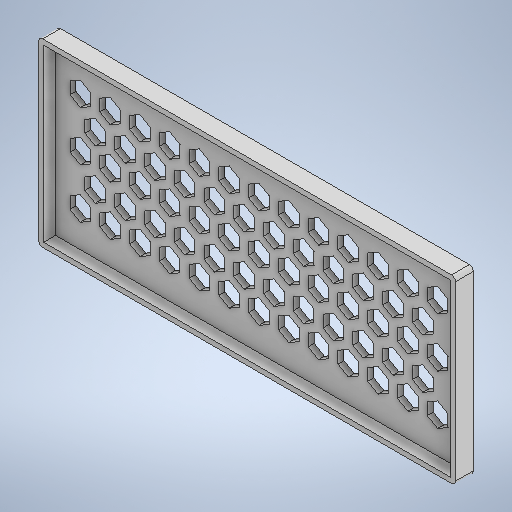
# Autodesk Inventor part: lm2596_box_lid_test
Saved by Autodesk Inventor 2025 (Build 290162000, 162)
## iProperties
Created: 2025-01-26
Part Number: lm2596_box_lid_test
Material: Všeobecné
Document SubType Name: Modeling
Designer: lukas
Density: 1 g/cm^3
Appearance: Výchozí
Author: lukas
## iProperties of the stored document lm2596_box_lid_3D tisk.ipt
Created: 2025-01-26
Part Number: lm2596_box_lid_3D tisk
Material: Všeobecné
Document SubType Name: Modeling
Designer: lukas
Density: 1 g/cm^3
Appearance: Výchozí
Author: lukas
Autodesk Inventor part; units mm, degrees
ref_plane "YZ Plane" through (0, 0, 0) normal (1, 0, 0) x (0, 1, 0)
ref_plane "XZ Plane" through (0, 0, 0) normal (0, 1, 0) x (-1, 0, 0)
ref_plane "XY Plane" through (0, 0, 0) normal (0, 0, 1) x (1, 0, 0)
sketch "Náčrt1" plane through (0, 0, 0) normal (0, 0, 1) x (1, 0, 0)
  line L0 (-105, 45.5) -> (105, 45.5)
  line L1 (105, 45.5) -> (105, -45.5)
  line L2 (105, -45.5) -> (-105, -45.5)
  line L3 (-105, -45.5) -> (-105, 45.5)
  line L4 (0, 63.7) -> (0, -63.7) projected
  line L5 (-147, 0) -> (147, 0) projected
  point P0 (0, 0)
  dimension "d0" = 210
  dimension "d1" = 91
  constraints: 8 end point, 2 parallel, 1 horizontal, 1 perpendicular, 2 other
  measures "d0" distance of L1.end L2.end
  measures "d1" distance of L0.end L1.end
extrude "Vysunutí1" add sketch "Náčrt1" along normal blind 3
sketch "Náčrt2" plane through (0, 0, 3) normal (0, 0, 1) x (1, 0, 0)
  line L0 (-105, 45.5) -> (-105, -45.5) projected
  line L1 (-105, -45.5) -> (105, -45.5) projected
  line L2 (105, -45.5) -> (105, 45.5) projected
  line L3 (105, 45.5) -> (-105, 45.5) projected
  line L4 (-164.5, 0) -> (164.5, 0) projected
  line L5 (0, -63.7) -> (0, 63.7) projected
  line L6 (-102.5, 43) -> (-102.5, -43)
  line L7 (-102.5, -43) -> (102.5, -43)
  line L8 (102.5, -43) -> (102.5, 43)
  line L9 (102.5, 43) -> (-102.5, 43)
  line L10 (-105, 45.5) -> (105, 45.5)
  line L11 (105, 45.5) -> (105, -45.5)
  line L12 (105, -45.5) -> (-105, -45.5)
  line L13 (-105, -45.5) -> (-105, 45.5)
  point P0 (0, 0)
  dimension "d5" = 2.5
  constraints: 16 end point, 2 parallel, 1 horizontal, 1 perpendicular, 3 other
  measures "d5" distance between parallel lines of L3 L9
extrude "Vysunutí2" add sketch "Náčrt2" along normal blind 6 contours L3 L5 L9 L6 L4 L0 | L4 L6 L7 L5 L1 L0 | L3 L2 L4 L8 L9 L5 | L5 L7 L8 L4 L2 L1
fillet "Zaoblení2" radius 2 4 edges at (105, -45.5, 4.5) (105, 45.5, 4.5) (-105, -45.5, 4.5) (-105, 45.5, 4.5)
sketch "Náčrt6" plane through (0, 0, 0) normal (0, 0, -1) x (-1, 0, 0)
  arc A0 (105, 43.5) -> (103, 45.5) centre (103, 43.5) ccw projected
  line L0 (-103, 45.5) -> (103, 45.5) projected
  arc A1 (-103, 45.5) -> (-105, 43.5) centre (-103, 43.5) ccw projected
  line L1 (-105, -43.5) -> (-105, 43.5) projected
  arc A2 (-105, -43.5) -> (-103, -45.5) centre (-103, -43.5) ccw projected
  line L2 (103, -45.5) -> (-103, -45.5) projected
  arc A3 (103, -45.5) -> (105, -43.5) centre (103, -43.5) ccw projected
  line L3 (105, 43.5) -> (105, -43.5) projected
  line L4 (0, -64.2799) -> (0, 64.2799) projected
  line L5 (-165.0799, 0) -> (165.0799, 0) projected
  line L6 (0, 6) -> (5.1962, 3)
  line L7 (5.1962, 3) -> (5.1962, -3)
  line L8 (5.1962, -3) -> (0, -6)
  line L9 (0, -6) -> (-5.1962, -3)
  line L10 (-5.1962, -3) -> (-5.1962, 3)
  line L11 (-5.1962, 3) -> (0, 6)
  line L12 (0, 0) -> (-2.5981, -4.5) construction
  line L13 (-7.5, -12.9904) -> (-10.0981, -17.4904) construction
  line L14 (-7.5, -18.9904) -> (-12.6962, -15.9904)
  line L15 (-12.6962, -15.9904) -> (-12.6962, -9.9904)
  line L16 (-2.3038, -9.9904) -> (-2.3038, -15.9904)
  line L17 (-12.6962, -9.9904) -> (-7.5, -6.9904)
  line L18 (-7.5, -6.9904) -> (-2.3038, -9.9904)
  line L19 (-2.3038, -15.9904) -> (-7.5, -18.9904)
  line L20 (-20.1962, 3) -> (-15, 6)
  line L21 (-15, 6) -> (-9.8038, 3)
  line L22 (-20.1962, -3) -> (-20.1962, 3)
  line L23 (-15, -6) -> (-20.1962, -3)
  line L24 (-9.8038, -3) -> (-15, -6)
  line L25 (-9.8038, 3) -> (-9.8038, -3)
  line L26 (9.8038, 3) -> (15, 6)
  line L27 (15, 6) -> (20.1962, 3)
  line L28 (9.8038, -3) -> (9.8038, 3)
  line L29 (15, -6) -> (9.8038, -3)
  line L30 (20.1962, -3) -> (15, -6)
  line L31 (20.1962, 3) -> (20.1962, -3)
  line L32 (-35.1962, 3) -> (-30, 6)
  line L33 (-30, 6) -> (-24.8038, 3)
  line L34 (-35.1962, -3) -> (-35.1962, 3)
  line L35 (-30, -6) -> (-35.1962, -3)
  line L36 (-24.8038, -3) -> (-30, -6)
  line L37 (-24.8038, 3) -> (-24.8038, -3)
  line L38 (24.8038, 3) -> (30, 6)
  line L39 (30, 6) -> (35.1962, 3)
  line L40 (24.8038, -3) -> (24.8038, 3)
  line L41 (30, -6) -> (24.8038, -3)
  line L42 (35.1962, -3) -> (30, -6)
  line L43 (35.1962, 3) -> (35.1962, -3)
  line L44 (-50.1962, 3) -> (-45, 6)
  line L45 (-45, 6) -> (-39.8038, 3)
  line L46 (-50.1962, -3) -> (-50.1962, 3)
  line L47 (-45, -6) -> (-50.1962, -3)
  line L48 (-39.8038, -3) -> (-45, -6)
  line L49 (-39.8038, 3) -> (-39.8038, -3)
  line L50 (39.8038, 3) -> (45, 6)
  line L51 (45, 6) -> (50.1962, 3)
  line L52 (39.8038, -3) -> (39.8038, 3)
  line L53 (45, -6) -> (39.8038, -3)
  line L54 (50.1962, -3) -> (45, -6)
  line L55 (50.1962, 3) -> (50.1962, -3)
  line L56 (-65.1962, 3) -> (-60, 6)
  line L57 (-60, 6) -> (-54.8038, 3)
  line L58 (-65.1962, -3) -> (-65.1962, 3)
  line L59 (-60, -6) -> (-65.1962, -3)
  line L60 (-54.8038, -3) -> (-60, -6)
  line L61 (-54.8038, 3) -> (-54.8038, -3)
  line L62 (54.8038, 3) -> (60, 6)
  line L63 (60, 6) -> (65.1962, 3)
  line L64 (54.8038, -3) -> (54.8038, 3)
  line L65 (60, -6) -> (54.8038, -3)
  line L66 (65.1962, -3) -> (60, -6)
  line L67 (65.1962, 3) -> (65.1962, -3)
  line L68 (-80.1962, 3) -> (-75, 6)
  line L69 (-75, 6) -> (-69.8038, 3)
  line L70 (-80.1962, -3) -> (-80.1962, 3)
  line L71 (-75, -6) -> (-80.1962, -3)
  line L72 (-69.8038, -3) -> (-75, -6)
  line L73 (-69.8038, 3) -> (-69.8038, -3)
  line L74 (69.8038, 3) -> (75, 6)
  line L75 (75, 6) -> (80.1962, 3)
  line L76 (69.8038, -3) -> (69.8038, 3)
  line L77 (75, -6) -> (69.8038, -3)
  line L78 (80.1962, -3) -> (75, -6)
  line L79 (80.1962, 3) -> (80.1962, -3)
  line L80 (-95.1962, 3) -> (-90, 6)
  line L81 (-90, 6) -> (-84.8038, 3)
  line L82 (-95.1962, -3) -> (-95.1962, 3)
  line L83 (-90, -6) -> (-95.1962, -3)
  line L84 (-84.8038, -3) -> (-90, -6)
  line L85 (-84.8038, 3) -> (-84.8038, -3)
  line L86 (84.8038, 3) -> (90, 6)
  line L87 (90, 6) -> (95.1962, 3)
  line L88 (84.8038, -3) -> (84.8038, 3)
  line L89 (90, -6) -> (84.8038, -3)
  line L90 (95.1962, -3) -> (90, -6)
  line L91 (95.1962, 3) -> (95.1962, -3)
  line L92 (7.5, -12.9904) -> (4.9019, -17.4904) construction
  line L93 (2.3038, -9.9904) -> (7.5, -6.9904)
  line L94 (2.3038, -15.9904) -> (2.3038, -9.9904)
  line L95 (7.5, -18.9904) -> (2.3038, -15.9904)
  line L96 (12.6962, -15.9904) -> (7.5, -18.9904)
  line L97 (7.5, -6.9904) -> (12.6962, -9.9904)
  line L98 (12.6962, -9.9904) -> (12.6962, -15.9904)
  line L99 (22.5, -12.9904) -> (19.9019, -17.4904) construction
  line L100 (17.3038, -9.9904) -> (22.5, -6.9904)
  line L101 (17.3038, -15.9904) -> (17.3038, -9.9904)
  line L102 (22.5, -18.9904) -> (17.3038, -15.9904)
  line L103 (27.6962, -15.9904) -> (22.5, -18.9904)
  line L104 (22.5, -6.9904) -> (27.6962, -9.9904)
  line L105 (27.6962, -9.9904) -> (27.6962, -15.9904)
  line L106 (37.5, -12.9904) -> (34.9019, -17.4904) construction
  line L107 (32.3038, -9.9904) -> (37.5, -6.9904)
  line L108 (32.3038, -15.9904) -> (32.3038, -9.9904)
  line L109 (37.5, -18.9904) -> (32.3038, -15.9904)
  line L110 (42.6962, -15.9904) -> (37.5, -18.9904)
  line L111 (37.5, -6.9904) -> (42.6962, -9.9904)
  line L112 (42.6962, -9.9904) -> (42.6962, -15.9904)
  line L113 (52.5, -12.9904) -> (49.9019, -17.4904) construction
  line L114 (47.3038, -9.9904) -> (52.5, -6.9904)
  line L115 (47.3038, -15.9904) -> (47.3038, -9.9904)
  line L116 (52.5, -18.9904) -> (47.3038, -15.9904)
  line L117 (57.6962, -15.9904) -> (52.5, -18.9904)
  line L118 (52.5, -6.9904) -> (57.6962, -9.9904)
  line L119 (57.6962, -9.9904) -> (57.6962, -15.9904)
  line L120 (67.5, -12.9904) -> (64.9019, -17.4904) construction
  line L121 (62.3038, -9.9904) -> (67.5, -6.9904)
  line L122 (62.3038, -15.9904) -> (62.3038, -9.9904)
  line L123 (67.5, -18.9904) -> (62.3038, -15.9904)
  line L124 (72.6962, -15.9904) -> (67.5, -18.9904)
  line L125 (67.5, -6.9904) -> (72.6962, -9.9904)
  line L126 (72.6962, -9.9904) -> (72.6962, -15.9904)
  line L127 (82.5, -12.9904) -> (79.9019, -17.4904) construction
  line L128 (77.3038, -9.9904) -> (82.5, -6.9904)
  line L129 (77.3038, -15.9904) -> (77.3038, -9.9904)
  line L130 (82.5, -18.9904) -> (77.3038, -15.9904)
  line L131 (87.6962, -15.9904) -> (82.5, -18.9904)
  line L132 (82.5, -6.9904) -> (87.6962, -9.9904)
  line L133 (87.6962, -9.9904) -> (87.6962, -15.9904)
  line L134 (-27.6962, -9.9904) -> (-22.5, -6.9904)
  line L135 (-22.5, -6.9904) -> (-17.3038, -9.9904)
  line L136 (-27.6962, -15.9904) -> (-27.6962, -9.9904)
  line L137 (-22.5, -12.9904) -> (-25.0981, -17.4904) construction
  line L138 (-22.5, -18.9904) -> (-27.6962, -15.9904)
  line L139 (-17.3038, -15.9904) -> (-22.5, -18.9904)
  line L140 (-17.3038, -9.9904) -> (-17.3038, -15.9904)
  line L141 (-42.6962, -9.9904) -> (-37.5, -6.9904)
  line L142 (-37.5, -6.9904) -> (-32.3038, -9.9904)
  line L143 (-42.6962, -15.9904) -> (-42.6962, -9.9904)
  line L144 (-37.5, -12.9904) -> (-40.0981, -17.4904) construction
  line L145 (-37.5, -18.9904) -> (-42.6962, -15.9904)
  line L146 (-32.3038, -15.9904) -> (-37.5, -18.9904)
  line L147 (-32.3038, -9.9904) -> (-32.3038, -15.9904)
  line L148 (-57.6962, -9.9904) -> (-52.5, -6.9904)
  line L149 (-52.5, -6.9904) -> (-47.3038, -9.9904)
  line L150 (-57.6962, -15.9904) -> (-57.6962, -9.9904)
  line L151 (-52.5, -12.9904) -> (-55.0981, -17.4904) construction
  line L152 (-52.5, -18.9904) -> (-57.6962, -15.9904)
  line L153 (-47.3038, -15.9904) -> (-52.5, -18.9904)
  line L154 (-47.3038, -9.9904) -> (-47.3038, -15.9904)
  line L155 (-72.6962, -9.9904) -> (-67.5, -6.9904)
  line L156 (-67.5, -6.9904) -> (-62.3038, -9.9904)
  line L157 (-72.6962, -15.9904) -> (-72.6962, -9.9904)
  line L158 (-67.5, -12.9904) -> (-70.0981, -17.4904) construction
  line L159 (-67.5, -18.9904) -> (-72.6962, -15.9904)
  line L160 (-62.3038, -15.9904) -> (-67.5, -18.9904)
  line L161 (-62.3038, -9.9904) -> (-62.3038, -15.9904)
  line L162 (-87.6962, -9.9904) -> (-82.5, -6.9904)
  line L163 (-82.5, -6.9904) -> (-77.3038, -9.9904)
  line L164 (-87.6962, -15.9904) -> (-87.6962, -9.9904)
  line L165 (-82.5, -12.9904) -> (-85.0981, -17.4904) construction
  line L166 (-82.5, -18.9904) -> (-87.6962, -15.9904)
  line L167 (-77.3038, -15.9904) -> (-82.5, -18.9904)
  line L168 (-77.3038, -9.9904) -> (-77.3038, -15.9904)
  line L169 (37.5, 18.0096) -> (42.6962, 15.0096)
  line L170 (32.3038, 15.0096) -> (37.5, 18.0096)
  line L171 (42.6962, 15.0096) -> (42.6962, 9.0096)
  line L172 (42.6962, 9.0096) -> (37.5, 6.0096)
  line L173 (37.5, 12.0096) -> (34.9019, 7.5096) construction
  line L174 (37.5, 6.0096) -> (32.3038, 9.0096)
  line L175 (32.3038, 9.0096) -> (32.3038, 15.0096)
  line L176 (-22.5, 18.0096) -> (-17.3038, 15.0096)
  line L177 (-12.6962, 15.0096) -> (-7.5, 18.0096)
  line L178 (-17.3038, 15.0096) -> (-17.3038, 9.0096)
  line L179 (-17.3038, 9.0096) -> (-22.5, 6.0096)
  line L180 (-7.5, 18.0096) -> (-2.3038, 15.0096)
  line L181 (-12.6962, 9.0096) -> (-12.6962, 15.0096)
  line L182 (-7.5, 12.0096) -> (-10.0981, 7.5096) construction
  line L183 (-7.5, 6.0096) -> (-12.6962, 9.0096)
  line L184 (-2.3038, 9.0096) -> (-7.5, 6.0096)
  line L185 (-2.3038, 15.0096) -> (-2.3038, 9.0096)
  line L186 (2.3038, 9.0096) -> (2.3038, 15.0096)
  line L187 (2.3038, 15.0096) -> (7.5, 18.0096)
  line L188 (7.5, 18.0096) -> (12.6962, 15.0096)
  line L189 (7.5, 12.0096) -> (4.9019, 7.5096) construction
  line L190 (12.6962, 9.0096) -> (7.5, 6.0096)
  line L191 (7.5, 6.0096) -> (2.3038, 9.0096)
  line L192 (22.5, 18.0096) -> (27.6962, 15.0096)
  line L193 (27.6962, 15.0096) -> (27.6962, 9.0096)
  line L194 (17.3038, 15.0096) -> (22.5, 18.0096)
  line L195 (27.6962, 9.0096) -> (22.5, 6.0096)
  line L196 (22.5, 12.0096) -> (19.9019, 7.5096) construction
  line L197 (22.5, 6.0096) -> (17.3038, 9.0096)
  line L198 (-57.6962, 9.0096) -> (-57.6962, 15.0096)
  line L199 (-52.5, 6.0096) -> (-57.6962, 9.0096)
  line L200 (-52.5, 12.0096) -> (-55.0981, 7.5096) construction
  line L201 (-57.6962, 15.0096) -> (-52.5, 18.0096)
  line L202 (12.6962, 15.0096) -> (12.6962, 9.0096)
  line L203 (17.3038, 9.0096) -> (17.3038, 15.0096)
  line L204 (52.5, 18.0096) -> (57.6962, 15.0096)
  line L205 (62.3038, 15.0096) -> (67.5, 18.0096)
  line L206 (62.3038, 9.0096) -> (62.3038, 15.0096)
  line L207 (67.5, 12.0096) -> (64.9019, 7.5096) construction
  line L208 (67.5, 6.0096) -> (62.3038, 9.0096)
  line L209 (47.3038, 15.0096) -> (52.5, 18.0096)
  line L210 (52.5, 12.0096) -> (49.9019, 7.5096) construction
  line L211 (57.6962, 9.0096) -> (52.5, 6.0096)
  line L212 (47.3038, 9.0096) -> (47.3038, 15.0096)
  line L213 (52.5, 6.0096) -> (47.3038, 9.0096)
  line L214 (57.6962, 15.0096) -> (57.6962, 9.0096)
  line L215 (67.5, 18.0096) -> (72.6962, 15.0096)
  line L216 (72.6962, 9.0096) -> (67.5, 6.0096)
  line L217 (77.3038, 15.0096) -> (82.5, 18.0096)
  line L218 (72.6962, 15.0096) -> (72.6962, 9.0096)
  line L219 (77.3038, 9.0096) -> (77.3038, 15.0096)
  line L220 (82.5, 18.0096) -> (87.6962, 15.0096)
  line L221 (82.5, 12.0096) -> (79.9019, 7.5096) construction
  line L222 (82.5, 6.0096) -> (77.3038, 9.0096)
  line L223 (87.6962, 15.0096) -> (87.6962, 9.0096)
  line L224 (87.6962, 9.0096) -> (82.5, 6.0096)
  line L225 (-22.5, 12.0096) -> (-25.0981, 7.5096) construction
  line L226 (-27.6962, 15.0096) -> (-22.5, 18.0096)
  line L227 (-22.5, 6.0096) -> (-27.6962, 9.0096)
  line L228 (-27.6962, 9.0096) -> (-27.6962, 15.0096)
  line L229 (-32.3038, 15.0096) -> (-32.3038, 9.0096)
  line L230 (-32.3038, 9.0096) -> (-37.5, 6.0096)
  line L231 (-37.5, 18.0096) -> (-32.3038, 15.0096)
  line L232 (-37.5, 12.0096) -> (-40.0981, 7.5096) construction
  line L233 (-42.6962, 15.0096) -> (-37.5, 18.0096)
  line L234 (-37.5, 6.0096) -> (-42.6962, 9.0096)
  line L235 (-42.6962, 9.0096) -> (-42.6962, 15.0096)
  line L236 (-47.3038, 15.0096) -> (-47.3038, 9.0096)
  line L237 (-47.3038, 9.0096) -> (-52.5, 6.0096)
  line L238 (-52.5, 18.0096) -> (-47.3038, 15.0096)
  line L239 (-82.5, 18.0096) -> (-77.3038, 15.0096)
  line L240 (-87.6962, 15.0096) -> (-82.5, 18.0096)
  line L241 (-77.3038, 9.0096) -> (-82.5, 6.0096)
  line L242 (-82.5, 12.0096) -> (-85.0981, 7.5096) construction
  line L243 (-87.6962, 9.0096) -> (-87.6962, 15.0096)
  line L244 (-82.5, 6.0096) -> (-87.6962, 9.0096)
  line L245 (-77.3038, 15.0096) -> (-77.3038, 9.0096)
  line L246 (-67.5, 18.0096) -> (-62.3038, 15.0096)
  line L247 (-62.3038, 15.0096) -> (-62.3038, 9.0096)
  line L248 (-72.6962, 15.0096) -> (-67.5, 18.0096)
  line L249 (-62.3038, 9.0096) -> (-67.5, 6.0096)
  line L250 (-67.5, 12.0096) -> (-70.0981, 7.5096) construction
  line L251 (-72.6962, 9.0096) -> (-72.6962, 15.0096)
  line L252 (-67.5, 6.0096) -> (-72.6962, 9.0096)
  line L253 (-45, 31) -> (-39.8038, 28)
  line L254 (-15, 19) -> (-20.1962, 22)
  line L255 (-20.1962, 28) -> (-15, 31)
  line L256 (-20.1962, 22) -> (-20.1962, 28)
  line L257 (-39.8038, 28) -> (-39.8038, 22)
  line L258 (-30, 31) -> (-24.8038, 28)
  line L259 (-35.1962, 22) -> (-35.1962, 28)
  line L260 (-24.8038, 28) -> (-24.8038, 22)
  line L261 (-24.8038, 22) -> (-30, 19)
  line L262 (-30, 19) -> (-35.1962, 22)
  line L263 (-35.1962, 28) -> (-30, 31)
  line L264 (-39.8038, 22) -> (-45, 19)
  line L265 (-45, 19) -> (-50.1962, 22)
  line L266 (-50.1962, 28) -> (-45, 31)
  line L267 (-50.1962, 22) -> (-50.1962, 28)
  line L268 (-65.1962, 28) -> (-60, 31)
  line L269 (-60, 31) -> (-54.8038, 28)
  line L270 (-65.1962, 22) -> (-65.1962, 28)
  line L271 (-54.8038, 22) -> (-60, 19)
  line L272 (-54.8038, 28) -> (-54.8038, 22)
  line L273 (-60, 19) -> (-65.1962, 22)
  line L274 (-80.1962, 28) -> (-75, 31)
  line L275 (-75, 31) -> (-69.8038, 28)
  line L276 (-80.1962, 22) -> (-80.1962, 28)
  line L277 (-69.8038, 28) -> (-69.8038, 22)
  line L278 (-69.8038, 22) -> (-75, 19)
  line L279 (-75, 19) -> (-80.1962, 22)
  line L280 (-84.8038, 28) -> (-84.8038, 22)
  line L281 (-90, 31) -> (-84.8038, 28)
  line L282 (-95.1962, 28) -> (-90, 31)
  line L283 (-95.1962, 22) -> (-95.1962, 28)
  line L284 (-84.8038, 22) -> (-90, 19)
  line L285 (-90, 19) -> (-95.1962, 22)
  line L286 (69.8038, 28) -> (75, 31)
  line L287 (69.8038, 22) -> (69.8038, 28)
  line L288 (60, 31) -> (65.1962, 28)
  line L289 (75, 19) -> (69.8038, 22)
  line L290 (65.1962, 28) -> (65.1962, 22)
  line L291 (54.8038, 28) -> (60, 31)
  line L292 (65.1962, 22) -> (60, 19)
  line L293 (54.8038, 22) -> (54.8038, 28)
  line L294 (50.1962, 28) -> (50.1962, 22)
  line L295 (35.1962, 22) -> (30, 19)
  line L296 (35.1962, 28) -> (35.1962, 22)
  line L297 (39.8038, 22) -> (39.8038, 28)
  line L298 (45, 19) -> (39.8038, 22)
  line L299 (-5.1962, 28) -> (0, 31)
  line L300 (-15, 31) -> (-9.8038, 28)
  line L301 (0, 31) -> (5.1962, 28)
  line L302 (-5.1962, 22) -> (-5.1962, 28)
  line L303 (-9.8038, 28) -> (-9.8038, 22)
  line L304 (-9.8038, 22) -> (-15, 19)
  line L305 (0, 25) -> (-2.5981, 20.5) construction
  line L306 (0, 19) -> (-5.1962, 22)
  line L307 (5.1962, 28) -> (5.1962, 22)
  line L308 (5.1962, 22) -> (0, 19)
  line L309 (9.8038, 28) -> (15, 31)
  line L310 (15, 31) -> (20.1962, 28)
  line L311 (24.8038, 22) -> (24.8038, 28)
  line L312 (24.8038, 28) -> (30, 31)
  line L313 (20.1962, 28) -> (20.1962, 22)
  line L314 (30, 31) -> (35.1962, 28)
  line L315 (39.8038, 28) -> (45, 31)
  line L316 (45, 31) -> (50.1962, 28)
  line L317 (50.1962, 22) -> (45, 19)
  line L318 (60, 19) -> (54.8038, 22)
  line L319 (80.1962, 22) -> (75, 19)
  line L320 (75, 31) -> (80.1962, 28)
  line L321 (90, 19) -> (84.8038, 22)
  line L322 (80.1962, 28) -> (80.1962, 22)
  line L323 (95.1962, 22) -> (90, 19)
  line L324 (84.8038, 22) -> (84.8038, 28)
  line L325 (84.8038, 28) -> (90, 31)
  line L326 (95.1962, 28) -> (95.1962, 22)
  line L327 (90, 31) -> (95.1962, 28)
  line L328 (9.8038, 22) -> (9.8038, 28)
  line L329 (15, 19) -> (9.8038, 22)
  line L330 (20.1962, 22) -> (15, 19)
  line L331 (30, 19) -> (24.8038, 22)
  line L332 (24.8038, -22) -> (30, -19)
  line L333 (15, -19) -> (20.1962, -22)
  line L334 (15, -31) -> (9.8038, -28)
  line L335 (9.8038, -28) -> (9.8038, -22)
  line L336 (9.8038, -22) -> (15, -19)
  line L337 (20.1962, -28) -> (15, -31)
  line L338 (20.1962, -22) -> (20.1962, -28)
  line L339 (24.8038, -28) -> (24.8038, -22)
  line L340 (30, -31) -> (24.8038, -28)
  line L341 (35.1962, -28) -> (30, -31)
  line L342 (39.8038, -28) -> (39.8038, -22)
  line L343 (39.8038, -22) -> (45, -19)
  line L344 (30, -19) -> (35.1962, -22)
  line L345 (35.1962, -22) -> (35.1962, -28)
  line L346 (45, -31) -> (39.8038, -28)
  line L347 (50.1962, -28) -> (45, -31)
  line L348 (50.1962, -22) -> (50.1962, -28)
  line L349 (54.8038, -22) -> (60, -19)
  line L350 (60, -19) -> (65.1962, -22)
  line L351 (75, -31) -> (69.8038, -28)
  line L352 (65.1962, -28) -> (60, -31)
  line L353 (69.8038, -28) -> (69.8038, -22)
  line L354 (65.1962, -22) -> (65.1962, -28)
  line L355 (54.8038, -28) -> (54.8038, -22)
  line L356 (60, -31) -> (54.8038, -28)
  line L357 (90, -31) -> (84.8038, -28)
  line L358 (95.1962, -28) -> (90, -31)
  line L359 (80.1962, -22) -> (80.1962, -28)
  line L360 (84.8038, -28) -> (84.8038, -22)
  line L361 (84.8038, -22) -> (90, -19)
  line L362 (95.1962, -22) -> (95.1962, -28)
  line L363 (90, -19) -> (95.1962, -22)
  line L364 (80.1962, -28) -> (75, -31)
  line L365 (75, -19) -> (80.1962, -22)
  line L366 (69.8038, -22) -> (75, -19)
  line L367 (45, -19) -> (50.1962, -22)
  line L368 (-50.1962, -22) -> (-45, -19)
  line L369 (-45, -19) -> (-39.8038, -22)
  line L370 (-54.8038, -22) -> (-54.8038, -28)
  line L371 (-50.1962, -28) -> (-50.1962, -22)
  line L372 (-39.8038, -22) -> (-39.8038, -28)
  line L373 (-45, -31) -> (-50.1962, -28)
  line L374 (-39.8038, -28) -> (-45, -31)
  line L375 (-65.1962, -28) -> (-65.1962, -22)
  line L376 (-80.1962, -22) -> (-75, -19)
  line L377 (-75, -19) -> (-69.8038, -22)
  line L378 (-69.8038, -22) -> (-69.8038, -28)
  line L379 (-69.8038, -28) -> (-75, -31)
  line L380 (-75, -31) -> (-80.1962, -28)
  line L381 (-80.1962, -28) -> (-80.1962, -22)
  line L382 (-65.1962, -22) -> (-60, -19)
  line L383 (-60, -19) -> (-54.8038, -22)
  line L384 (-95.1962, -22) -> (-90, -19)
  line L385 (-90, -19) -> (-84.8038, -22)
  line L386 (-95.1962, -28) -> (-95.1962, -22)
  line L387 (-90, -31) -> (-95.1962, -28)
  line L388 (-84.8038, -28) -> (-90, -31)
  line L389 (-84.8038, -22) -> (-84.8038, -28)
  line L390 (-54.8038, -28) -> (-60, -31)
  line L391 (-60, -31) -> (-65.1962, -28)
  line L392 (-24.8038, -28) -> (-30, -31)
  line L393 (-30, -31) -> (-35.1962, -28)
  line L394 (-20.1962, -22) -> (-15, -19)
  line L395 (-15, -31) -> (-20.1962, -28)
  line L396 (0, -19) -> (5.1962, -22)
  line L397 (5.1962, -22) -> (5.1962, -28)
  line L398 (0, -25) -> (-2.5981, -29.5) construction
  line L399 (5.1962, -28) -> (0, -31)
  line L400 (-5.1962, -28) -> (-5.1962, -22)
  line L401 (0, -31) -> (-5.1962, -28)
  line L402 (-5.1962, -22) -> (0, -19)
  line L403 (-9.8038, -22) -> (-9.8038, -28)
  line L404 (-9.8038, -28) -> (-15, -31)
  line L405 (-15, -19) -> (-9.8038, -22)
  line L406 (-20.1962, -28) -> (-20.1962, -22)
  line L407 (-24.8038, -22) -> (-24.8038, -28)
  line L408 (-30, -19) -> (-24.8038, -22)
  line L409 (-35.1962, -28) -> (-35.1962, -22)
  line L410 (-35.1962, -22) -> (-30, -19)
  point P0 (-15, 0)
  point P1 (-17.5981, -4.5)
  point P2 (15, 0)
  point P3 (12.4019, -4.5)
  point P4 (-30, 0)
  point P5 (-32.5981, -4.5)
  point P6 (30, 0)
  point P7 (27.4019, -4.5)
  point P8 (-45, 0)
  point P9 (-47.5981, -4.5)
  point P10 (45, 0)
  point P11 (42.4019, -4.5)
  point P12 (-60, 0)
  point P13 (-62.5981, -4.5)
  point P14 (60, 0)
  point P15 (57.4019, -4.5)
  point P16 (-75, 0)
  point P17 (-77.5981, -4.5)
  point P18 (75, 0)
  point P19 (72.4019, -4.5)
  point P20 (-90, 0)
  point P21 (-92.5981, -4.5)
  point P22 (90, 0)
  point P23 (87.4019, -4.5)
  point P24 (-37.5, 31.0096)
  point P25 (-40.0981, 32.5096)
  point P26 (-45, 25)
  point P27 (-17.5981, 20.5)
  point P28 (-15, 25)
  point P29 (-25.0981, 32.5096)
  point P30 (-22.5, 31.0096)
  point P31 (-30, 25)
  point P32 (-32.5981, 20.5)
  point P33 (-47.5981, 20.5)
  point P34 (-60, 25)
  point P35 (-55.0981, 32.5096)
  point P36 (-52.5, 31.0096)
  point P37 (-62.5981, 20.5)
  point P38 (-70.0981, 32.5096)
  point P39 (-67.5, 31.0096)
  point P40 (-75, 25)
  point P41 (-82.5, 31.0096)
  point P42 (-85.0981, 32.5096)
  point P43 (-77.5981, 20.5)
  point P44 (-90, 25)
  point P45 (-92.5981, 20.5)
  point P46 (75, 25)
  point P47 (72.4019, 20.5)
  point P48 (60, 25)
  point P49 (-7.5, 31.0096)
  point P50 (-10.0981, 32.5096)
  point P51 (4.9019, 32.5096)
  point P52 (7.5, 31.0096)
  point P53 (45, 25)
  point P54 (42.4019, 20.5)
  point P55 (22.5, 31.0096)
  point P56 (19.9019, 32.5096)
  point P57 (30, 25)
  point P58 (34.9019, 32.5096)
  point P59 (37.5, 31.0096)
  point P60 (52.5, 31.0096)
  point P61 (49.9019, 32.5096)
  point P62 (57.4019, 20.5)
  point P63 (79.9019, 32.5096)
  point P64 (67.5, 31.0096)
  point P65 (64.9019, 32.5096)
  point P66 (82.5, 31.0096)
  point P67 (87.4019, 20.5)
  point P68 (90, 25)
  point P69 (15, 25)
  point P70 (12.4019, 20.5)
  point P71 (27.4019, 20.5)
  point P72 (12.4019, -29.5)
  point P73 (15, -25)
  point P74 (27.4019, -29.5)
  point P75 (30, -25)
  point P76 (45, -25)
  point P77 (42.4019, -29.5)
  point P78 (37.5, -31.9904)
  point P79 (60, -25)
  point P80 (67.5, -31.9904)
  point P81 (72.4019, -29.5)
  point P82 (75, -25)
  point P83 (57.4019, -29.5)
  point P84 (87.4019, -29.5)
  point P85 (90, -25)
  point P86 (7.5, -31.9904)
  point P87 (22.5, -31.9904)
  point P88 (82.5, -31.9904)
  point P89 (52.5, -31.9904)
  point P90 (-45, -25)
  point P91 (-47.5981, -29.5)
  point P92 (-75, -25)
  point P93 (-77.5981, -29.5)
  point P94 (-60, -25)
  point P95 (-90, -25)
  point P96 (-92.5981, -29.5)
  point P97 (-52.5, -31.9904)
  point P98 (-62.5981, -29.5)
  point P99 (-67.5, -31.9904)
  point P100 (-82.5, -31.9904)
  point P101 (-32.5981, -29.5)
  point P102 (-37.5, -31.9904)
  point P103 (-17.5981, -29.5)
  point P104 (-22.5, -31.9904)
  point P105 (-7.5, -31.9904)
  point P106 (-15, -25)
  point P107 (-30, -25)
  dimension "d62" = 6
  dimension "d65" = 15
  dimension "d72" = 15
  dimension "d79" = 15
  dimension "d86" = 15
  dimension "d110" = 25
  dimension "d117" = 25
  dimension "d124" = 25
  constraints: 810 end point, 3 horizontal, 3 vertical, 1 coincident, 1 collinear, 1 midpoint, 1 point on line, 968 other
  measures "d62" distance of L6.end L7.end
  measures "d65" distance of L12.end L13.end
  measures "d72" distance of L12.start point (-15, 0)
  measures "d79" distance of L14.start L95.start
  measures "d86" distance of L17.end L134.end
  measures "d110" distance of L107.end L169.start
  measures "d117" distance of L230.end point (-37.5, 31.01)
  measures "d124" distance of L230.end point (-37.5, -18.99)
extrude "Vysunutí6" cut sketch "Náčrt6" against normal blind 10 contours L91 L90 L89 L88 L5 | L5 L88 L86 L87 L91 | L301 L307 L308 L4 | L4 L306 L302 L299 | L79 L78 L77 L76 L5 | L5 L76 L74 L75 L79 | L6 L7 L5 L4 | L4 L5 L10 L11 | L401 L400 L402 L4 | L4 L396 L397 L399 | L82 L80 L81 L85 L5 | L5 L85 L84 L83 L82 | L5 L7 L8 L4 | L4 L9 L10 L5 | L67 L66 L65 L64 L5 | L5 L64 L62 L63 L67 | L70 L68 L69 L73 L5 | L5 L73 L72 L71 L70 | L25 L24 L23 L22 L5 | L5 L22 L20 L21 L25 | L28 L26 L27 L31 L5 | L5 L31 L30 L29 L28 | L55 L54 L53 L52 L5 | L5 L52 L50 L51 L55 | L58 L56 L57 L61 L5 | L5 L61 L60 L59 L58 | L37 L36 L35 L34 L5 | L5 L34 L32 L33 L37 | L40 L38 L39 L43 L5 | L5 L43 L42 L41 L40 | L46 L44 L45 L49 L5 | L5 L49 L48 L47 L46 | L14 L15 L17 L18 L16 L19 | L93 L97 L98 L96 L95 L94 | L100 L104 L105 L103 L102 L101 | L107 L111 L112 L110 L109 L108 | L114 L118 L119 L117 L116 L115 | L121 L125 L126 L124 L123 L122 | L128 L132 L133 L131 L130 L129 | L134 L135 L140 L139 L138 L136 | L141 L142 L147 L146 L145 L143 | L148 L149 L154 L153 L152 L150 | L155 L156 L161 L160 L159 L157 | L162 L163 L168 L167 L166 L164 | L169 L171 L172 L174 L175 L170 | L176 L178 L179 L227 L228 L226 | L177 L180 L185 L184 L183 L181 | L186 L187 L188 L202 L190 L191 | L192 L193 L195 L197 L203 L194 | L198 L201 L238 L236 L237 L199 | L204 L214 L211 L213 L212 L209 | L205 L215 L218 L216 L208 L206 | L217 L220 L223 L224 L222 L219 | L229 L230 L234 L235 L233 L231 | L239 L245 L241 L244 L243 L240 | L246 L247 L249 L252 L251 L248 | L253 L257 L264 L265 L267 L266 | L254 L256 L255 L300 L303 L304 | L258 L260 L261 L262 L259 L263 | L268 L269 L272 L271 L273 L270 | L274 L275 L277 L278 L279 L276 | L280 L284 L285 L283 L282 L281 | L286 L320 L322 L319 L289 L287 | L288 L290 L292 L318 L293 L291 | L294 L317 L298 L297 L315 L316 | L295 L331 L311 L312 L314 L296 | L309 L310 L313 L330 L329 L328 | L321 L324 L325 L327 L326 L323 | L332 L344 L345 L341 L340 L339 | L333 L338 L337 L334 L335 L336 | L342 L343 L367 L348 L347 L346 | L349 L350 L354 L352 L356 L355 | L351 L353 L366 L365 L359 L364 | L357 L360 L361 L363 L362 L358 | L368 L369 L372 L374 L373 L371 | L370 L390 L391 L375 L382 L383 | L376 L377 L378 L379 L380 L381 | L384 L385 L389 L388 L387 L386 | L392 L393 L409 L410 L408 L407 | L394 L405 L403 L404 L395 L406
